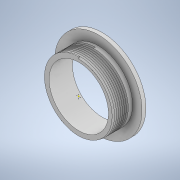
# Autodesk Inventor part: laserseal
Saved by Autodesk Inventor 2022.2 (Build 262287030, 287C)
## iProperties
Created: 2022-05-17
Part Number: laserseal
Material: Generic
Document SubType Name: Modeling
Designer: Tapendra
Density: 1 g/cm^3
Appearance: Default
Author: Tapendra
Autodesk Inventor part; units mm, degrees
ref_plane "XZ Plane" through (0, 0, 0) normal (0, 1, 0) x (-1, 0, 0)
ref_plane "XY Plane" through (0, 0, 0) normal (0, 0, 1) x (1, 0, 0)
sketch "Sketch1" plane through (0, 0, 0) normal (0, 0, 1) x (1, 0, 0)
  circle A0 centre (0, 0) radius 15.2
  circle A1 centre (0, 0) radius 22.37
  dimension "d0" = 30.4
  dimension "d1" = 44.74
  constraints: 2 centre point, 2 coincident
  measures "d0" diameter of A0
  measures "d1" diameter of A1
extrude "Extrusion1" add sketch "Sketch1" along normal blind 2
sketch "Sketch2" plane through (0, 0, 2) normal (0, 0, 1) x (1, 0, 0)
  circle A0 centre (0, 0) radius 15.2
  circle A1 centre (0, 0) radius 22.37 projected
  circle A2 centre (0, 0) radius 17.565
  circle A3 centre (0, 0) radius 15.2 projected
  dimension "d4" = 35.13
  constraints: 2 centre point, 2 coincident, 1 concentric
  measures "d4" diameter of A2
extrude "Extrusion2" add sketch "Sketch2" along normal blind 10 contours A2
sketch "Sketch3" plane through (0, 0, 12) normal (0, 0, 1) x (1, 0, 0)
  point P0 (0, 0)
  point P1 (0, 0)
  constraints: 1 coincident
ref_plane "Work Plane1" through (0, 0, 0) normal (1, 0, 0) x (0, 1, 0)
sketch "Sketch4" plane through (0, 0, 0) normal (1, 0, 0) x (0, 1, 0)
  line L0 (17.565, 12) -> (-17.565, 12) projected
  line L1 (0, 12) -> (0, 0) construction
  line L2 (-15.2, 0) -> (15.2, 0) projected
  line L3 (17.565, 12.5095) -> (16.565, 12)
  line L4 (16.565, 12) -> (17.565, 11.4905)
  line L5 (17.565, 11.4905) -> (17.565, 12.5095)
  line L6 (17.565, 2) -> (17.565, 12) construction
  line L7 (17.565, 10.2903) -> (17.565, 3.7005)
  dimension "d8" = 0
  dimension "d9" = 0
  dimension "d10" = 1
  constraints: 10 end point, 2 point on line, 1 equal length, 1 midpoint, 1 parallel, 1 perpendicular
  measures "d8" distance between parallel lines of L6 L5
  measures "d9" distance from line of L0 L3.end
  measures "d10" distance from line of L3.end L5
coil "Coil1" sketch "Sketch4" operation cut axis through (0, 0, 12) along (0, 0, -1) pitch 1 turns 8 hand right
body "Solid1"
